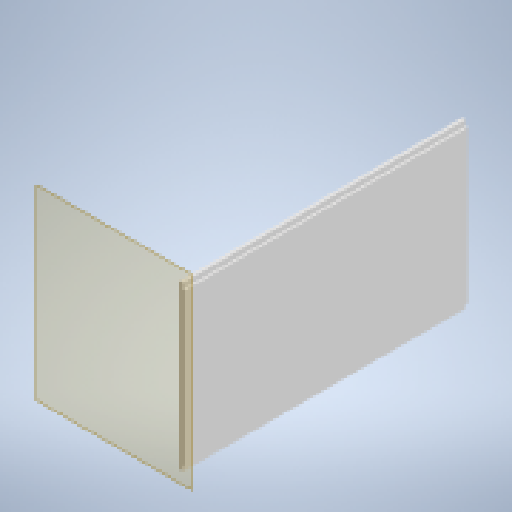
# Autodesk Inventor part: Lid1
Saved by Autodesk Inventor 2026 (Build 300175050, 175E)
## iProperties
Created: 2025-08-01
Part Number: Lid1
Material: Plastic, Opaque White
Document SubType Name: Sheet Metal
Designer: Cupri
Mass: 167.504 g
Surface Area: 762.076 cm^2
Volume: 175.95 cm^3
Density: 0.952 g/cm^3
Sheet Metal Rule: Default
Appearance: Smooth - White
Author: Cupri
Autodesk Inventor part; units mm, degrees
ref_plane "YZ Plane" through (0, 0, 0) normal (1, 0, 0) x (0, 1, 0)
ref_plane "XZ Plane" through (0, 0, 0) normal (0, 1, 0) x (-1, 0, 0)
ref_plane "XY Plane" through (0, 0, 0) normal (0, 0, 1) x (1, 0, 0)
ref_plane "Work Plane1" through (0, 0, 0) normal (0, 0, 1) x (1, 0, 0)
sketch "Sketch1" plane through (0, 0, 0) normal (0, 0, 1) x (1, 0, 0)
  line L0 (62.538, -67.5) -> (62.538, 67.5) projected
  line L1 (60.7565, 80) -> (90.6942, 80) projected
  line L2 (57.538, 75) -> (57.538, -75) projected
  line L3 (60.538, 72.3) -> (57.538, 72.3) projected
  line L4 (60.538, 67.5) -> (60.538, 72.5) projected
  line L5 (60.538, -72.3) -> (57.538, -72.3) projected
  line L6 (60.538, -72.5) -> (60.538, -67.5) projected
  line L7 (62.538, -67.5) -> (60.538, -67.5) projected
  line L8 (57.538, 72.3) -> (60.538, 72.3)
  line L9 (60.538, 72.3) -> (60.538, -72.3)
  line L10 (60.538, -72.3) -> (57.538, -72.3)
  line L11 (57.538, -72.3) -> (57.538, 72.3)
  line L12 (62.538, -67.5) -> (60.538, -67.5)
  line L13 (60.538, -67.5) -> (60.538, 67.5)
  line L14 (60.538, 67.5) -> (62.538, 67.5)
  line L15 (62.538, 67.5) -> (62.538, -67.5)
  point P0 (0, 0)
  constraints: 16 end point, 4 parallel, 2 horizontal, 2 perpendicular
ref_plane "Work Plane2" through (-62.538, -75, -250) normal (0, 0, 1) x (1, 0, 0)
extrude "Extrusion1" add sketch "Sketch1" against normal up to surface (250 mm away)
equation "\"BendRadius\" = Thickness"
equation "\"BendReliefWidth\" = Thickness"
equation "\"BendReliefDepth\" = 0.5 * Thickness"
equation "\"CornerReliefSize\" = 4 * Thickness"
equation "\"MinimumRemnant\" = 2 * Thickness"
equation "\"TransitionRadius\" = BendRadius"
equation "\"JacobiRadiusSize\" = BendRadius"
equation "\"GapSize\" = Thickness"
equation "\"Thickness\" = 3.048"
body "Solid1"
